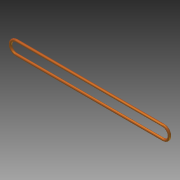
# Autodesk Inventor part: uptake polycord
Saved by Autodesk Inventor 2012 (Build 160160000, 160)
## iProperties
Created: 2013-07-07
Part Number: uptake polycord
Material: Default
Document SubType Name: Modeling
Designer: Bryce
Density: 1 g/cm^3
Author: Bryce
Autodesk Inventor part; units mm, degrees
ref_plane "YZ Plane" through (0, 0, 0) normal (1, 0, 0) x (0, 1, 0)
ref_plane "XZ Plane" through (0, 0, 0) normal (0, 1, 0) x (-1, 0, 0)
ref_plane "XY Plane" through (0, 0, 0) normal (0, 0, 1) x (1, 0, 0)
sketch "Sketch1" plane through (0, 0, 0) normal (0, 0, 1) x (1, 0, 0)
  arc A0 (0, 15.875) -> (0, -15.875) centre (0, 0) ccw
  line L0 (0, 15.875) -> (384.175, 15.875)
  arc A1 (384.175, -15.875) -> (384.175, 15.875) centre (384.175, 0) ccw
  line L1 (384.175, -15.875) -> (0, -15.875)
  dimension "d0" = 384.175
  dimension "d1" = 15.875
  constraints: 4 end point, 4 point on circle, 4 tangent, 2 centre point, 1 coincident, 1 horizontal, 1 parallel
  measures "d0" distance of L0.start L0.end
  measures "d1" radius of A0
sketch "Sketch2" plane through (0, 0, 0) normal (1, 0, 0) x (0, 1, 0)
  circle A0 centre (15.875, 0) radius 3.175
  point P0 (0, 0)
  dimension "d2" = 15.875
  dimension "d3" = 6.35
  constraints: 1 centre point, 1 horizontal alignment
  measures "d2" distance of point (0, 0) A0.centre
  measures "d3" diameter of A0
sweep "Sweep1" add profiles "Sketch2" path "Sketch1"
body "Solid1"
